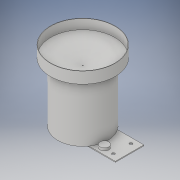
# Autodesk Inventor part: pluviometro
Saved by Autodesk Inventor 2019.4 (Build 234330000, 330)
## iProperties
Created: 2021-02-17
Part Number: pluviometro
Material: Genérico
Document SubType Name: Modeling
Designer: Lattes
Density: 1 g/cm^3
Appearance: Padrão
Author: Lattes
Autodesk Inventor part; units mm, degrees
ref_plane "YZ Plane" through (0, 0, 0) normal (1, 0, 0) x (0, 1, 0)
ref_plane "XZ Plane" through (0, 0, 0) normal (0, 1, 0) x (-1, 0, 0)
ref_plane "XY Plane" through (0, 0, 0) normal (0, 0, 1) x (1, 0, 0)
sketch "Esboço2" plane through (0, 0, 0) normal (0, 0, 1) x (1, 0, 0)
  line L0 (0, 0) -> (57, 0)
  line L1 (57, 0) -> (57, 125)
  line L2 (74, 135) -> (74, 161)
  line L3 (74, 161) -> (73, 161)
  line L4 (57, 125) -> (74, 135)
  line L5 (73, 135.5719) -> (56, 125.5719)
  line L6 (56, 125.5719) -> (56, 1)
  line L7 (56, 1) -> (1, 1)
  line L8 (1, 1) -> (0, 1)
  line L9 (0, 1) -> (0, 0)
  line L10 (0, 45.3298) -> (0, 108.1085)
  line L11 (73, 160) -> (73, 161)
  line L12 (73, 138.8946) -> (0.9659, 119.5931)
  line L13 (73, 138.8946) -> (148.5752, 138.8946) construction
  line L14 (0.9659, 118.5931) -> (73, 137.8946)
  line L15 (73, 160) -> (73, 138.8946)
  line L16 (73, 137.8946) -> (73, 135.5719)
  line L17 (0.9659, 119.5931) -> (0.9659, 118.5931)
  dimension "d0" = 57
  dimension "d1" = 125
  dimension "d5" = 26
  dimension "d8" = 1
  dimension "d9" = 165
  constraints: 36 end point, 5 perpendicular, 3 horizontal, 2 vertical, 1 parallel, 2 other
  measures "d0" distance of L0.start L0.end
  measures "d1" distance of L0.end L1.end
  measures "d5" distance of L2.start L2.end
  measures "d8" distance of L7.end L8.end
  measures "d9" angle of L12 L13
revolve "Revolução1" add sketch "Esboço2" angle 360 about axis through (0, 45.3298, 0) along (0, 1, 0)
sketch "Esboço3" plane through (0, 0, 0) normal (0, -1, 0) x (1, 0, 0)
  circle A0 centre (0, 0) radius 2.5
  dimension "d13" = 5
  constraints: 1 centre point, 1 coincident
  measures "d13" diameter of A0
extrude "Extrusão1" cut sketch "Esboço3" against normal blind 10
sketch "Esboço4" plane through (0, 0, 0) normal (0, -1, 0) x (1, 0, 0)
  circle A0 centre (0, 0) radius 57 projected
  line L0 (107, 0) -> (107, 32.5)
  line L1 (107, 32.5) -> (107, -32.5)
  line L2 (107, -32.5) -> (27, -32.5)
  line L3 (27, -32.5) -> (107, -32.5)
  line L4 (107, -32.5) -> (107, 32.5)
  line L5 (107, 32.5) -> (27, 32.5)
  line L6 (27, 32.5) -> (27, -32.5)
  point P0 (0, 0)
  dimension "d17" = 32.5
  dimension "d18" = 65
  dimension "d19" = 80
  constraints: 14 end point, 2 parallel, 2 perpendicular, 1 horizontal, 1 point on line
  measures "d17" distance of L0.start L0.end
  measures "d18" distance of L0.end L1.end
  measures "d19" distance of L1.end L2.end
extrude "Extrusão2" add sketch "Esboço4" along normal blind 2 contours A0 L2 L6 L5 | A0 L5 L0 L1 L2 picked at (37, 0)
sketch "Esboço5" plane through (27, 0, 32.5) normal (0, -1, 0) x (1, 0, 0)
  circle A0 centre (-27, -32.5) radius 2.5 projected
  line L0 (-27, -32.5) -> (-65, -32.5)
  circle A1 centre (-65, -32.5) radius 2.5
  dimension "d22" = 38
  dimension "d23" = 5
  constraints: 2 end point, 1 centre point, 1 coincident, 1 horizontal
  measures "d22" distance of L0.start L0.end
  measures "d23" diameter of A1
extrude "Extrusão3" cut sketch "Esboço5" along normal mid plane 6 contours A1
pattern_circular "Padrão circular1" count 4 over 360 about axis through (0, 0, 0) along (0, 1, 0) of "Extrusão3"
sketch "Esboço6" plane through (0, -2, 0) normal (0, -1, 0) x (1, 0, 0)
  line L0 (107, -32.5) -> (107, 32.5) projected
  line L1 (107, 0) -> (90, 0)
  line L2 (90, 0) -> (90, 20)
  line L3 (90, 0) -> (90, -20)
  circle A0 centre (90, -20) radius 3.25
  circle A1 centre (90, 20) radius 3.25
  point P0 (0, 0)
  dimension "d29" = 17
  dimension "d30" = 20
  dimension "d31" = 20
  dimension "d32" = 6.5
  dimension "d33" = 6.5
  constraints: 6 end point, 2 centre point, 2 coincident, 1 horizontal, 1 midpoint, 1 perpendicular, 1 vertical
  measures "d29" distance of L1.start L1.end
  measures "d30" distance of L1.end L2.end
  measures "d31" distance of L1.end L3.end
  measures "d32" diameter of A0
  measures "d33" diameter of A1
extrude "Extrusão4" cut sketch "Esboço6" against normal blind 6
sketch "Esboço7" plane through (0, 0, 0) normal (0, 1, 0) x (1, 0, 0)
  arc A0 (46.8268, -32.5) -> (46.8268, 32.5) centre (0, 0) ccw projected
  line L0 (57, 0) -> (57, -32.5)
  line L1 (46.8268, -32.5) -> (107, -32.5) projected
  line L2 (57, 0) -> (89.5, 0) construction
  line L3 (57, -32.5) -> (57, -27.5)
  line L4 (57, -27.5) -> (77, -27.5)
  line L5 (77, -27.5) -> (77, -17.5)
  line L6 (77, -17.5) -> (67, -17.5)
  circle A1 centre (67, -17.5) radius 10
  point P0 (0, 0)
  dimension "d36" = 90
  dimension "d37" = 5
  dimension "d38" = 20
  dimension "d39" = 10
  dimension "d40" = 10
  constraints: 12 end point, 4 perpendicular, 2 point on line, 1 centre point, 1 coincident, 1 horizontal, 1 point on circle, 1 tangent
  measures "d36" angle of L0 L2
  measures "d37" distance of L0.end L3.end
  measures "d38" distance of L3.end L4.end
  measures "d39" distance of L4.end L5.end
  measures "d40" distance of L5.end L6.end
extrude "Extrusão5" add sketch "Esboço7" along normal blind 6 contours A1
